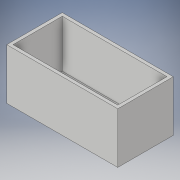
# Autodesk Inventor part: enclosure
Saved by Autodesk Inventor 2018 (Build 220112000, 112)
## iProperties
Created: 2018-03-12
Part Number: enclosure
Material: Generic
Document SubType Name: Modeling
Designer: Josh
Density: 1 g/cm^3
Appearance: Default
Author: Josh
Autodesk Inventor part; units mm, degrees
ref_plane "YZ Plane" through (0, 0, 0) normal (1, 0, 0) x (0, 1, 0)
ref_plane "XZ Plane" through (0, 0, 0) normal (0, 1, 0) x (-1, 0, 0)
ref_plane "Work Plane1" through (-43.4917, 1.5875, -7.62) normal (0, -1, 0) x (1, 0, 0)
sketch "Sketch3" plane through (-43.4917, 1.5875, -7.62) normal (0, -1, 0) x (1, 0, 0)
  line L0 (-106.9189, -23.7145) -> (70.8811, -23.7145)
  line L1 (70.8811, -23.7145) -> (70.8811, 65.1855)
  line L2 (70.8811, 65.1855) -> (-106.9189, 65.1855)
  line L3 (-106.9189, 65.1855) -> (-106.9189, -23.7145)
  line L4 (-106.9189, -23.7145) -> (70.8811, -23.7145)
  line L5 (70.8811, -23.7145) -> (70.8811, -18.6345)
  line L6 (70.8811, -18.6345) -> (-106.9189, -18.6345)
  line L7 (-106.9189, -18.6345) -> (-106.9189, -23.7145)
  line L8 (-106.9189, 65.1855) -> (-101.8389, 65.1855)
  line L9 (-101.8389, 65.1855) -> (-101.8389, -23.7145)
  line L10 (-101.8389, -23.7145) -> (-106.9189, -23.7145)
  line L11 (-106.9189, -23.7145) -> (-106.9189, 65.1855)
  line L12 (-106.9189, 65.1855) -> (70.8811, 65.1855)
  line L13 (70.8811, 65.1855) -> (70.8811, 60.1055)
  line L14 (70.8811, 60.1055) -> (-106.9189, 60.1055)
  line L15 (-106.9189, 60.1055) -> (-106.9189, 65.1855)
  line L16 (70.8811, -23.7145) -> (65.8011, -23.7145)
  line L17 (65.8011, -23.7145) -> (65.8011, 65.1855)
  line L18 (65.8011, 65.1855) -> (70.8811, 65.1855)
  line L19 (70.8811, 65.1855) -> (70.8811, -23.7145)
  point P0 (43.4917, 7.62)
  dimension "d1" = 177.8
  dimension "d2" = 88.9
  dimension "d3" = 5.08
  dimension "d4" = 5.08
  dimension "d5" = 5.08
  dimension "d6" = 5.08
  constraints: 40 end point, 10 parallel, 5 horizontal, 5 perpendicular, 4 point on line
  measures "d1" distance of L2.end L1.end
  measures "d2" distance of L1.end L0.end
  measures "d3" distance of L5.end L4.end
  measures "d4" distance of L9.end L10.end
  measures "d5" distance of L12.end L13.end
  measures "d6" distance of L17.end L18.end
extrude "Extrusion1" add sketch "Sketch3" against normal blind 76.2 contours L3 L2 L9 L14 | L9 L2 L17 L14 | L17 L2 L1 L14
extrude "Extrusion2" cut sketch "Sketch3" against normal blind 76.2 contours L3 L6 L9 L0 | L3 L14 L9 L6 | L3 L2 L9 L14
extrude "Extrusion3" cut sketch "Sketch3" against normal blind 76.2 contours L3 L6 L9 L0 | L9 L6 L17 L0 | L3 L14 L9 L6 | L17 L6 L1 L0 | L3 L2 L9 L14 | L17 L14 L1 L6 | L17 L2 L1 L14
extrude "Extrusion4" add sketch "Sketch3" against normal blind 76.2 contours L3 L6 L9 L0 | L3 L14 L9 L6 | L3 L2 L9 L14
extrude "Extrusion5" add sketch "Sketch3" against normal blind 76.2 contours L17 L6 L1 L0 | L17 L14 L1 L6 | L17 L2 L1 L14
extrude "Extrusion6" add sketch "Sketch3" against normal blind 76.2 contours L3 L6 L9 L0 | L9 L6 L17 L0 | L17 L6 L1 L0
extrude "Extrusion7" add sketch "Sketch3" along normal blind 5.08 contours L9 L14 L17 L6
extrude "Extrusion8" add sketch "Sketch3" along normal blind 5.08 contours L17 L6 L1 L0 | L17 L14 L1 L6 | L17 L2 L1 L14
extrude "Extrusion9" add sketch "Sketch3" along normal blind 5.08 contours L3 L6 L9 L0 | L9 L6 L17 L0 | L17 L6 L1 L0
extrude "Extrusion10" add sketch "Sketch3" along normal blind 5.08 contours L3 L6 L9 L0 | L3 L14 L9 L6 | L3 L2 L9 L14
extrude "Extrusion11" add sketch "Sketch3" along normal blind 5.08 contours L3 L2 L9 L14 | L9 L2 L17 L14 | L17 L2 L1 L14
body "Solid1"
